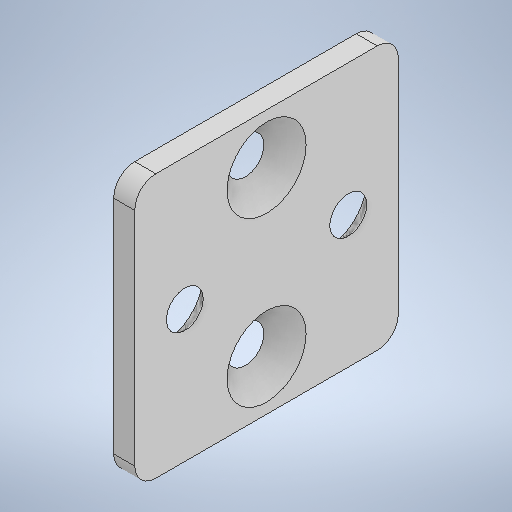
# Autodesk Inventor part: TRILHO FRONTAL
Saved by Autodesk Inventor 2025.2 (Build 292293000, 293)
## iProperties
Created: 2025-05-14
Part Number: TRILHO FRONTAL
Material: Genérico
Document SubType Name: Modeling
Designer: marce
Density: 1 g/cm^3
Appearance: Padrão
Author: marce
Autodesk Inventor part; units mm, degrees
ref_plane "YZ Plane" through (0, 0, 0) normal (1, 0, 0) x (0, 1, 0)
ref_plane "XZ Plane" through (0, 0, 0) normal (0, 1, 0) x (-1, 0, 0)
ref_plane "XY Plane" through (0, 0, 0) normal (0, 0, 1) x (1, 0, 0)
sketch "Esboço1" plane through (0, 0, 0) normal (1, 0, 0) x (0, 1, 0)
  line L0 (0, 0) -> (25, 0)
  line L1 (25, 0) -> (25, -25)
  line L2 (25, -25) -> (0, -25)
  line L3 (0, -25) -> (0, 0)
  dimension "d0" = 25
  dimension "d1" = 25
  constraints: 8 end point, 2 parallel, 1 horizontal, 1 perpendicular
  measures "d0" distance of L1.end L2.end
  measures "d1" distance of L0.end L1.end
extrude "Extrusão1" add sketch "Esboço1" along normal blind 2
fillet "Arredondamento1" radius 2 1 edges at (1, 25, 0)
fillet "Arredondamento2" radius 2 1 edges at (1, 0, 0)
fillet "Arredondamento3" radius 2 1 edges at (1, 25, -25)
fillet "Arredondamento4" radius 2 1 edges at (1, 0, -25)
sketch "Esboço2" plane through (2, 0, 0) normal (1, 0, 0) x (0, 0, -1)
  line L0 (23, 25) -> (2, 25) projected
  line L1 (2, 0) -> (23, 0) projected
  line L2 (0, 23) -> (0, 2) projected
  line L3 (0, 12.5) -> (4.75, 12.5)
  line L4 (25, 2) -> (25, 23) projected
  line L5 (25, 12.5) -> (20.25, 12.5)
  point P0 (0, 0)
  point P1 (12.5, 20.25)
  point P2 (12.5, 4.75)
  dimension "d11" = 4.75
  dimension "d12" = 4.75
  constraints: 4 end point, 2 coincident, 2 horizontal, 2 midpoint
  measures "d11" distance of L3.start L3.end
  measures "d12" distance of L5.start L5.end
hole "Furo1" at (2, 20.25, -12.5) at (2, 4.75, -12.5) direction (-1, 0, 0) diameter 3.242 depth 4 countersink diameter 7.5 countersink angle 90 thread size "M4x0.7" class "6H" standard "ANSI Metric M Profile"
sketch "Esboço3" plane through (0, 0, 0) normal (-1, 0, 0) x (0, 0, 1)
  line L0 (-25, 2) -> (-25, 23) projected
  line L1 (-25, 12.5) -> (-20.25, 12.5)
  line L2 (0, 23) -> (0, 2) projected
  line L3 (0, 12.5) -> (-4.75, 12.5)
  point P0 (0, 0)
  dimension "d20" = 4.75
  dimension "d21" = 4.75
  constraints: 4 end point, 2 coincident, 2 horizontal, 2 midpoint
  measures "d20" distance of L1.start L1.end
  measures "d21" distance of L3.start L3.end
hole "Furo2" at (0, 12.5, -20.25) at (0, 12.5, -4.75) direction (1, 0, 0) diameter 3.242 depth 4 countersink diameter 7.5 countersink angle 90 thread size "M4x0.7" class "6H" standard "ANSI Metric M Profile"
